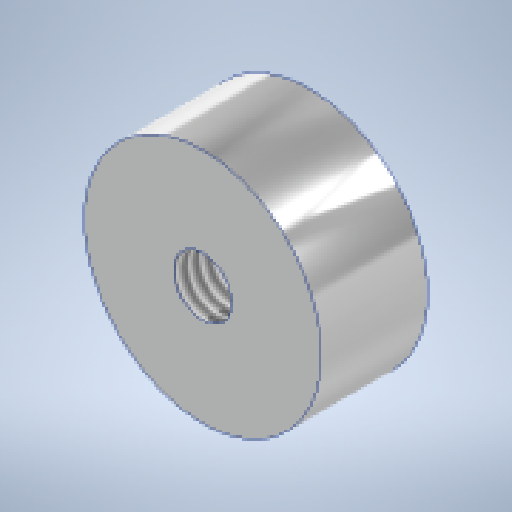
# Autodesk Inventor part: shortshaft2
Saved by Autodesk Inventor 2024.3 (Build 283343010, 343A)
## iProperties
Created: 2026-03-07
Part Number: shortshaft2
Material: アルミニウム 6061
Document SubType Name: Modeling
Designer: kshau
Density: 2.7 g/cm^3
Appearance: アルミニウム - フラット
Author: kshau
Autodesk Inventor part; units mm, degrees
ref_plane "YZ Plane" through (0, 0, 0) normal (1, 0, 0) x (0, 1, 0)
ref_plane "XZ Plane" through (0, 0, 0) normal (0, 1, 0) x (-1, 0, 0)
ref_plane "XY Plane" through (0, 0, 0) normal (0, 0, 1) x (1, 0, 0)
sketch "スケッチ1" plane through (0, 0, 0) normal (0, 0, 1) x (1, 0, 0)
  circle A0 centre (0, 0) radius 5
  dimension "d0" = 10
  constraints: 1 centre point, 1 coincident
  measures "d0" diameter of A0
extrude "押し出し1" add sketch "スケッチ1" along normal blind 4.5
sketch "スケッチ2" plane through (0, 0, 0) normal (0, 0, -1) x (-1, 0, 0)
  circle A0 centre (0, 0) radius 5 projected
  constraints: 1 coincident
hole "穴1" at (0, 0, 0) direction (0, 0, 1) diameter 2.459 depth 10 thread size "M3x0.5" class "6H" standard "ISO Metric profile"
